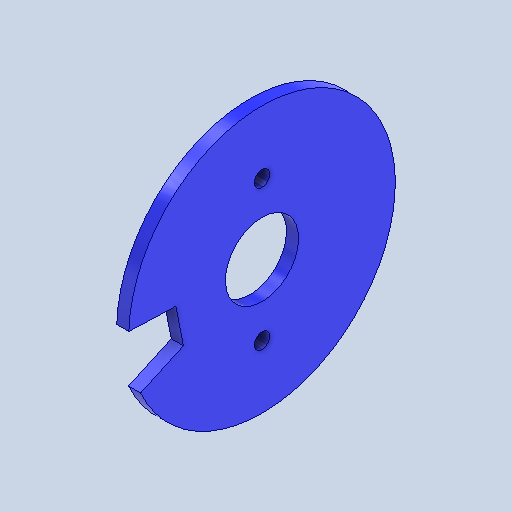
# Autodesk Inventor part: belt_liner_v3_3DP_P-1-F
Saved by Autodesk Inventor 2025.2 (Build 292293000, 293)
## iProperties
Created: 2025-01-19
Part Number: belt_liner_v3_3DP_P-1-F
Material: ABS プラスチック
Document SubType Name: Modeling
Designer: haruy
Density: 1.06 g/cm^3
Appearance: 青 - 壁塗料 - 光沢
Author: haruy
Autodesk Inventor part; units mm, degrees
ref_plane "YZ Plane" through (0, 0, 0) normal (1, 0, 0) x (0, 1, 0)
ref_plane "XZ Plane" through (0, 0, 0) normal (0, 1, 0) x (-1, 0, 0)
ref_plane "XY Plane" through (0, 0, 0) normal (0, 0, 1) x (1, 0, 0)
sketch "スケッチ1" plane through (0, 0, 0) normal (1, 0, 0) x (0, 1, 0)
  line L0 (6.5943, 27.3747) -> (6.2554, 17.6758)
  line L1 (6.2554, 17.6758) -> (-1.5909, 16.1151)
  line L2 (-1.5909, 16.1151) -> (-5.6155, 24.946)
  arc A0 (-5.6155, 24.946) -> (6.5943, 27.3747) centre (5.7151, -0.1112) ccw
  circle A1 centre (5.7151, -0.1112) radius 7.55
  circle A2 centre (-8.7849, -0.1112) radius 1.6
  circle A3 centre (20.2151, -0.1112) radius 1.6
  point P0 (0, 0)
  constraints: 6 end point, 4 centre point, 2 point on circle
extrude "押し出し1" add sketch "スケッチ1" along normal blind 2.5
